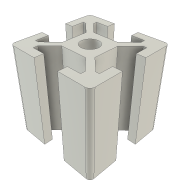
# Autodesk Inventor part: Aluminium profile 20x20 6mm slot
Saved by Autodesk Inventor 2018 (Build 220112000, 112)
## iProperties
Created: 2019-03-18
Part Number: Aluminium profile 20x20 6mm slot
Material: Generic
Document SubType Name: Modeling
Designer: Paolo Minieri
Density: 1 g/cm^3
Appearance: Default
Mass: 3.65725 g
Surface Area: 38.2816 cm^2
Volume: 3.65725 cm^3
Author: Paolo Minieri
Autodesk Inventor part; units mm, degrees
ref_plane "YZ Plane" through (0, 0, 0) normal (1, 0, 0) x (0, 1, 0)
ref_plane "XZ Plane" through (0, 0, 0) normal (0, 1, 0) x (-1, 0, 0)
ref_plane "XY Plane" through (0, 0, 0) normal (0, 0, 1) x (1, 0, 0)
sketch "Schizzo1" plane through (0, 0, 0) normal (0, 0, 1) x (1, 0, 0)
  arc A0 (36.9231, 17.4874) -> (37.9231, 18.4874) centre (36.9231, 18.4874) ccw
  line L0 (27.9231, 37.356) -> (27.9231, 17.6188) construction
  line L1 (36.9231, 17.4874) -> (30.9231, 17.4874)
  line L2 (30.9231, 19.4874) -> (33.9231, 19.4874)
  line L3 (30.9231, 19.4874) -> (30.9231, 17.4874)
  line L4 (33.9231, 19.4874) -> (33.9231, 20.5217)
  line L5 (35.9231, 21.4874) -> (35.1213, 21.4874)
  line L6 (33.9231, 20.5217) -> (30.9273, 23.4874)
  line L7 (31.958, 23.6188) -> (32.4267, 23.6188) construction
  line L8 (35.1213, 21.4874) -> (31.9231, 24.6188)
  line L9 (27.9231, 28.7445) -> (27.9203, 28.7473)
  line L10 (27.9231, 27.4874) -> (16.785, 27.4874) construction
  line L11 (35.9231, 21.4874) -> (35.9231, 24.4874)
  line L12 (35.9231, 24.4874) -> (37.9231, 24.4874)
  line L13 (37.9231, 24.4874) -> (37.9231, 18.4874)
  line L14 (0.5417, 54.5893) -> (0.5417, -0.7152) construction
  arc A1 (17.9231, 18.4874) -> (18.9231, 17.4874) centre (18.9231, 18.4874) ccw
  line L15 (18.9231, 17.4874) -> (24.9231, 17.4874)
  line L16 (24.9231, 19.4874) -> (21.9231, 19.4874)
  line L17 (24.9231, 19.4874) -> (24.9231, 17.4874)
  line L18 (21.9231, 19.4874) -> (21.9231, 20.5217)
  line L19 (19.9231, 21.4874) -> (20.725, 21.4874)
  line L20 (21.9231, 20.5217) -> (24.919, 23.4874)
  line L21 (23.958, 23.6188) -> (23.9231, 23.6188) construction
  line L22 (19.9231, 21.4874) -> (19.9231, 24.4874)
  line L23 (19.9231, 24.4874) -> (17.9231, 24.4874)
  line L24 (17.9231, 24.4874) -> (17.9231, 18.4874)
  line L25 (33.8225, 24.3529) -> (33.8225, 24.4874)
  arc A2 (37.9231, 36.4874) -> (36.9231, 37.4874) centre (36.9231, 36.4874) ccw
  line L26 (36.9231, 37.4874) -> (30.9231, 37.4874)
  line L27 (30.9231, 35.4874) -> (33.9231, 35.4874)
  line L28 (30.9231, 35.4874) -> (30.9231, 37.4874)
  line L29 (33.9231, 35.4874) -> (33.9231, 34.4531)
  line L30 (35.9231, 33.4874) -> (35.1213, 33.4874)
  line L31 (33.9231, 34.4531) -> (30.9273, 31.4874)
  line L32 (31.958, 31.356) -> (32.4267, 31.356) construction
  line L33 (35.1213, 33.4874) -> (31.9231, 30.356)
  line L34 (35.9231, 33.4874) -> (35.9231, 30.4874)
  line L35 (35.9231, 30.4874) -> (37.9231, 30.4874)
  line L36 (37.9231, 30.4874) -> (37.9231, 36.4874)
  arc A3 (18.9231, 37.4874) -> (17.9231, 36.4874) centre (18.9231, 36.4874) ccw
  line L37 (19.9231, 30.4874) -> (17.9231, 30.4874)
  line L38 (19.9231, 33.4874) -> (20.725, 33.4874)
  line L39 (19.9231, 33.4874) -> (19.9231, 30.4874)
  line L40 (21.9231, 34.4531) -> (24.919, 31.4874)
  line L41 (24.9231, 35.4874) -> (21.9231, 35.4874)
  line L42 (21.9231, 35.4874) -> (21.9231, 34.4531)
  line L43 (24.9231, 35.4874) -> (24.9231, 37.4874)
  line L44 (18.9231, 37.4874) -> (24.9231, 37.4874)
  line L45 (17.9231, 30.4874) -> (17.9231, 36.4874)
  line L46 (33.8225, 30.6219) -> (33.8225, 30.4874)
  line L47 (30.9273, 23.4874) -> (24.919, 23.4874)
  line L48 (23.9231, 24.549) -> (23.9231, 30.4259)
  line L49 (24.919, 31.4874) -> (30.9273, 31.4874)
  line L50 (31.9231, 30.356) -> (31.9231, 24.6188)
  line L51 (23.9231, 24.549) -> (20.725, 21.4874)
  line L52 (23.9231, 30.4259) -> (20.725, 33.4874)
  circle A4 centre (27.9231, 27.4874) radius 2.1
  point P0 (0, 0)
  point P1 (17.9231, 17.6188)
  point P2 (22.0237, 24.3529)
  point P3 (24.8821, 25.7341)
  point P4 (23.4196, 23.6188)
  point P5 (17.9231, 37.356)
  point P6 (22.0237, 30.6219)
  point P7 (24.8821, 29.2408)
  point P8 (27.958, 27.4874)
  dimension "d104" = 20
  dimension "d111" = 8
  dimension "d112" = 4.2
  dimension "d115" = 20
  dimension "d116" = 6
  dimension "d117" = 4
  dimension "d118" = 1
  dimension "d119" = 12
  dimension "d129" = 6
  dimension "d130" = 6
  dimension "d131" = 6
  dimension "d132" = 2
  dimension "d133" = 2
  dimension "d134" = 2
  dimension "d135" = 2
  dimension "d136" = 12
  dimension "d137" = 12
  dimension "d146" = 8
  constraints: 104 end point, 45 symmetric about line, 8 point on circle, 5 centre point, 5 perpendicular, 4 horizontal, 4 point on line, 3 vertical, 2 parallel, 1 coincident, 1 midpoint, 1 tangent, 3 other
  measures "d104" distance between parallel lines of L36 L45
  measures "d111" distance between parallel lines of L48 L50
  measures "d112" diameter of A4
  measures "d115" distance between parallel lines of L15 L44
  measures "d116" distance between parallel lines of L23 L37
  measures "d117" distance between parallel lines of L48 L39
  measures "d118" radius of A0
  measures "d119" distance between parallel lines of L19 L38
  measures "d129" distance between parallel lines of L28 L43
  measures "d130" distance between parallel lines of L12 L35
  measures "d131" distance between parallel lines of L3 L17
  measures "d132" distance of L23.start L23.end
  measures "d133" distance of L37.start L45.start
  measures "d134" distance of L41.start L43.end
  measures "d135" distance of L27.start L26.end
  measures "d136" distance between parallel lines of L5 L30
  measures "d137" distance between parallel lines of L29 L42
  measures "d146" distance between parallel lines of L47 L49
extrude "Estrusione1" add sketch "Schizzo1" along normal blind 20
